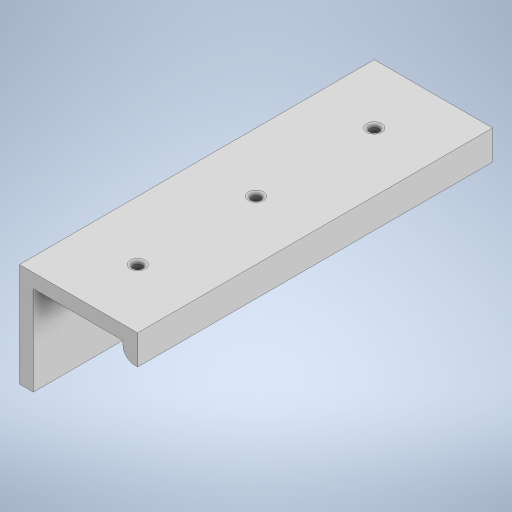
# Autodesk Inventor part: Block Bracket Mark Guide Tool
Saved by Autodesk Inventor 2023 (Build 270158000, 158)
## iProperties
Created: 2023-01-09
Part Number: Block Bracket Mark Guide Tool
Material: Generic
Document SubType Name: Modeling
Designer: justi
Density: 1 g/cm^3
Appearance: Default
Author: justi
Autodesk Inventor part; units mm, degrees
ref_plane "YZ Plane" through (0, 0, 0) normal (1, 0, 0) x (0, 1, 0)
ref_plane "XZ Plane" through (0, 0, 0) normal (0, 1, 0) x (-1, 0, 0)
ref_plane "XY Plane" through (0, 0, 0) normal (0, 0, 1) x (1, 0, 0)
sketch "Sketch9" plane through (0, 0, 0) normal (0, 1, 0) x (-1, 0, 0)
  line L0 (0, 0) -> (19.05, 0)
  line L1 (19.05, 0) -> (19.05, -76.2)
  line L2 (19.05, -76.2) -> (0, -76.2)
  line L3 (0, -76.2) -> (0, 0)
  circle A0 centre (9.525, -38.1) radius 0.9922
  circle A1 centre (9.525, -12.7) radius 0.9922
  circle A2 centre (9.525, -63.5) radius 0.9922
  dimension "d41" = 76.2
  dimension "d42" = 19.05
  dimension "d43" = 1.9844
  dimension "d44" = 9.525
  dimension "d45" = 38.1
  dimension "d46" = 1.9844
  dimension "d47" = 1.9844
  dimension "d48" = 9.525
  dimension "d49" = 9.525
  dimension "d50" = 25.4
  dimension "d51" = 25.4
  constraints: 8 end point, 3 centre point, 2 parallel, 1 horizontal, 1 perpendicular
  measures "d41" distance of L0.end L1.end
  measures "d42" distance of L1.end L2.end
  measures "d43" diameter of A0
  measures "d44" distance from line of L1 A0.centre
  measures "d45" distance from line of L2 A0.centre
  measures "d46" diameter of A1
  measures "d47" diameter of A2
  measures "d48" distance from line of L3 A1.centre
  measures "d49" distance from line of L3 A2.centre
  measures "d50" distance of A1.centre A0.centre
  measures "d51" distance of A2.centre A0.centre
extrude "Extrusion7" add sketch "Sketch9" along normal blind 3.175
sketch "Sketch10" plane through (0, 3.175, 0) normal (0, 1, 0) x (1, 0, 0)
  line L0 (-19.05, 76.2) -> (-19.05, 0) projected
  line L1 (-19.05, 0) -> (-22.225, 0)
  line L2 (-22.225, 0) -> (-22.225, 76.2)
  line L3 (-22.225, 76.2) -> (-19.05, 76.2)
  line L4 (-19.05, 76.2) -> (-19.05, 0)
  point P0 (0, 0)
  dimension "d54" = 3.175
  dimension "d55" = 76.2
  constraints: 8 end point, 2 parallel, 1 horizontal, 1 perpendicular
  measures "d54" distance of L2.end L3.end
  measures "d55" distance of L1.end L2.end
extrude "Extrusion8" add sketch "Sketch10" against normal blind 22.225
sketch "Sketch11" plane through (-19.05, 0, 0) normal (1, 0, 0) x (0, 0, -1)
  circle A0 centre (25.4, -9.525) radius 0.9922
  circle A1 centre (50.8, -9.525) radius 0.9922
  line L0 (76.2, -19.05) -> (0, -19.05) projected
  line L1 (0, 0) -> (0, -19.05) projected
  dimension "d58" = 1.9844
  dimension "d59" = 1.9844
  dimension "d60" = 9.525
  dimension "d61" = 9.525
  dimension "d62" = 25.4
  dimension "d63" = 25.4
  constraints: 2 centre point
  measures "d58" diameter of A0
  measures "d59" diameter of A1
  measures "d60" distance from line of L0 A0.centre
  measures "d61" distance from line of L0 A1.centre
  measures "d62" distance of A1.centre A0.centre
  measures "d63" distance from line of L1 A0.centre
extrude "Extrusion9" cut sketch "Sketch11" against normal blind 22.225
sketch "Sketch12" plane through (0, 0, 0) normal (0, 0, 1) x (1, 0, 0)
  line L0 (-19.05, 0) -> (-19.05, -19.05) projected
  line L1 (-19.05, 0) -> (-19.2296, 0.1796)
  line L2 (-19.05, 0) -> (0, 0) projected
  line L3 (-19.2296, 0.1796) -> (0, 0.1796)
  line L4 (0, 0.1796) -> (0, -19.05)
  line L5 (0, -19.05) -> (-19.2296, -19.05)
  line L6 (-19.2296, -19.05) -> (-19.2296, 0.1796)
  point P0 (0, 0)
  dimension "d68" = 0.254
  dimension "d69" = 135
  constraints: 10 end point, 2 parallel, 1 horizontal, 1 perpendicular, 1 point on line
  measures "d68" distance of L0.start L1.end
  measures "d69" angle of L2 L1
extrude "Extrusion10" cut sketch "Sketch12" against normal blind 76.2
fillet "Fillet4" radius 0.635 5 edges at (-22.225, -9.525, -24.4078) (-22.225, -9.525, -49.8078) (-8.5328, 3.175, -63.5) (-8.5328, 3.175, -38.1) (-8.5328, 3.175, -12.7)
sketch "Sketch13" plane through (0, 3.175, -76.2) normal (0, 0, -1) x (-1, 0, 0)
  line L0 (22.225, 0) -> (0, 0) projected
  line L1 (0, 0) -> (-3.175, 0)
  line L2 (-3.175, 0) -> (-3.175, -6.35)
  line L3 (-3.175, -6.35) -> (0, -6.35)
  line L4 (0, -6.35) -> (0, 0)
  point P0 (0, -3.175)
  dimension "d73" = 3.175
  dimension "d74" = 6.35
  constraints: 8 end point, 2 parallel, 1 horizontal, 1 perpendicular
  measures "d73" distance of L0.end L1.end
  measures "d74" distance of L1.end L2.end
extrude "Extrusion11" add sketch "Sketch13" against normal blind 76.2
fillet "Fillet5" radius 2.54 1 edges at (0, -3.175, -38.1)
body "Solid2"
